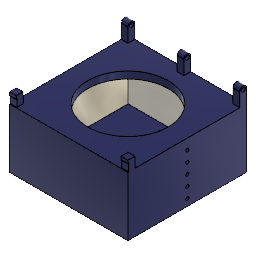
Final N95 UV Storage Container - Box v16 (Autodesk Fusion 360 design; units mm, degrees)
Autodesk Fusion 360 part; units mm, degrees
note: some values were not read from the file. Set by a fixed rule: which sketch regions a step uses.
sketch "Sketch1" plane through (0, 0, 0) normal (0, 0, 1) x (1, 0, 0)
  line L0 (0, 0) -> (170, 0)
  line L1 (170, 0) -> (170, 170)
  line L2 (170, 170) -> (0, 170)
  line L3 (0, 170) -> (0, 0)
  line L4 (0, 0) -> (85, 85)
  line L5 (87.25, 82.75) -> (82.75, 82.75)
  line L6 (82.75, 82.75) -> (82.75, 87.25)
  line L7 (82.75, 87.25) -> (87.25, 87.25)
  line L8 (87.25, 87.25) -> (87.25, 82.75)
  line L9 (87.25, 82.75) -> (82.75, 87.25) construction
  line L10 (82.75, 82.75) -> (87.25, 87.25) construction
  circle A0 centre (85, 85) radius 1.5
  point P0 (85, 85)
  dimension "d2" = 170
  dimension "d3" = 170
  dimension "d22" = 4.5
  dimension "d23" = 4.5
  dimension "d24" = 3
  dimension "d85" = 0
  dimension "d86" = 0
  dimension "d87" = 0
  dimension "d88" = 0
  dimension "d105" = 0
  dimension "d106" = 0
  dimension "d107" = 0
  dimension "d108" = 0
  dimension "d165" = 0
  dimension "d166" = 0
  dimension "d167" = 0
  dimension "d168" = 0
  dimension "d173" = 0
  dimension "d174" = 0
  dimension "d175" = 0
  dimension "d176" = 0
  dimension "d181" = 0
  dimension "d182" = 0
  dimension "d183" = 0
  constraint horizontal L0
  constraint vertical L1
  constraint horizontal L2
  constraint vertical L3
  constraint coincident L0.start L3.end
  constraint horizontal L5
  constraint perpendicular L5 L6
  constraint parallel L5 L7
  constraint parallel L6 L8
  constraint coincident L9 P0
  constraint coincident L10 P0
  constraint coincident P0 L4.end
  measures "d2" distance of L0.start L0.end
  measures "d3" distance of L0.start L2.end
  measures "d22" distance of L6.end L7.end
  measures "d23" distance of L5.end L6.end
  measures "d24" diameter of A0
extrude "Extrude1" add sketch "Sketch1" along normal blind 85 contours L0 L1 L2 L3 | L5 L6 L7 L8 | A0 makes body 1
shell "Shell1" thickness 10 removed faces 1 at (56.6667, 113.3333, 85) on bodies 1
extrude "Extrude3" cut sketch "Sketch1" along normal through all contours A0 bodies 1
extrude "Extrude4" cut sketch "Sketch1" along normal blind 10 and the other way blind -8 contours L5 L6 L7 L8 bodies 1
sketch "Sketch2" plane through (0, 0, 85) normal (0, 0, 1) x (-1, 0, 0)
  line L0 (-10, -160) -> (-160, -160)
  line L1 (-160, -160) -> (-160, -10)
  line L2 (-160, -10) -> (-10, -10)
  line L3 (-10, -10) -> (-10, -160)
  line L4 (0, -170) -> (0, 0)
  line L5 (0, 0) -> (-170, 0)
  line L6 (-170, 0) -> (-170, -170)
  line L7 (-170, -170) -> (0, -170)
  line L8 (0, -170) -> (-170, -170)
  line L9 (-170, -170) -> (-170, 0)
  line L10 (-170, 0) -> (0, 0)
  line L11 (0, 0) -> (0, -170)
  line L12 (0, 0) -> (-85, -85)
  circle A0 centre (-85, -85) radius 57.5
  dimension "d7" = 115
  constraint horizontal L8
  constraint vertical L9
  constraint horizontal L10
  constraint vertical L11
  constraint coincident L5.end L6.start
  constraint coincident L4.start L7.end
  constraint coincident L4.end L5.start
  constraint coincident L12.end A0.centre
  measures "d7" diameter of A0
extrude "Extrude2" add sketch "Sketch2" against normal blind 10 contours L0 L1 L2 L3 bodies 1
sketch "Sketch3" plane through (0, 0, 0) normal (-1, 0, 0) x (0, -1, 0)
  line L0 (-170, 0) -> (0, 0)
  line L1 (0, 0) -> (0, 85)
  line L2 (0, 85) -> (-170, 85)
  line L3 (-170, 85) -> (-170, 0)
  line L4 (-85, 85) -> (-85, 40)
  line L5 (-85, 85) -> (-85, 55)
  line L6 (-85, 85) -> (-85, 25)
  line L7 (-85, 85) -> (-85, 10)
  line L8 (-85, 85) -> (-85, 70)
  circle A0 centre (-85, 70) radius 2.25
  circle A1 centre (-85, 55) radius 2.25
  circle A2 centre (-85, 40) radius 2.25
  circle A3 centre (-85, 25) radius 2.25
  circle A4 centre (-85, 10) radius 2.25
  dimension "d10" = 45
  dimension "d69" = 30
  dimension "d70" = 60
  dimension "d71" = 75
  dimension "d72" = 15
  dimension "d73" = 4.5
  dimension "d74" = 4.5
  dimension "d75" = 4.5
  dimension "d76" = 4.5
  dimension "d77" = 4.5
  constraint midpoint L2 L4.start
  constraint perpendicular L0 L4
  constraint perpendicular L2 L5
  constraint perpendicular L2 L6
  constraint parallel L6 L7
  constraint parallel L6 L8
  constraint coincident L8.end A0.centre
  constraint coincident L5.end A1.centre
  constraint coincident L4.end A2.centre
  constraint coincident L6.end A3.centre
  constraint coincident L7.end A4.centre
  measures "d10" distance of L4.start L4.end
  measures "d69" distance of L4.start L5.end
  measures "d70" distance of L4.start L6.end
  measures "d71" distance of L4.start L7.end
  measures "d72" distance of L4.start L8.end
  measures "d73" diameter of A0
  measures "d74" diameter of A1
  measures "d75" diameter of A2
  measures "d76" diameter of A3
  measures "d77" diameter of A4
extrude "Extrude10" cut sketch "Sketch3" against normal blind 5 contours L4 L5 L6 L7 L8 A0 | L4 L5 L6 L7 L8 A0 | L4 L5 L6 L7 A1 | L4 L5 L6 L7 A1 | L4 L6 L7 A2 | L4 L6 L7 A2 | L6 L7 A3 | L6 L7 A3 | A4 bodies 1
ref_plane "WorkPlane1" through (85, 85, 42.5) normal (0, -1, 0) x (1, 0, 0)
sketch "Sketch4" plane through (85, 85, 55) normal (0, -1, 0) x (1, 0, 0)
  line L0 (-85, 10) -> (-94.9989, 10.1458)
  line L1 (-94.9989, 10.1458) -> (-95.1448, 0.1469)
  point P0 (-85, 10)
  dimension "d13" = 10
  dimension "d14" = 10
  constraint coincident P0 L0.start
  constraint perpendicular L0 L1
  measures "d13" distance of P0 L0.end
  measures "d14" distance of L0.end L1.end
pipe "Pipe1" [suppressed]
ref_plane "WorkPlane2" through (85, 85, 42.5) normal (-1, 0, 0) x (0, -1, 0)
mirror "Mirror2" about plane through (85, 85, 42.5) normal (-1, 0, 0) of "Extrude10"
mirror "Mirror1" [suppressed]
sketch "Sketch6" plane through (170, 0, 0) normal (1, 0, 0) x (0, 1, 0)
  line L0 (0, 0) -> (170, 0)
  line L1 (170, 0) -> (170, 85)
  line L2 (170, 85) -> (0, 85)
  line L3 (0, 85) -> (0, 0)
  line L4 (170, 85) -> (160, 85)
  line L5 (160, 85) -> (160, 105)
  line L6 (160, 105) -> (170, 105)
  line L7 (170, 105) -> (170, 85)
  circle A0 centre (165, 105) radius 5
  line L8 (0, 85) -> (10, 85)
  line L9 (10, 85) -> (10, 100)
  line L10 (10, 100) -> (0, 100)
  line L11 (0, 100) -> (0, 85)
  circle A1 centre (165, 105) radius 3
  line L12 (0, 100) -> (0, 95)
  line L13 (0, 95) -> (1.0607, 96.0607)
  line L14 (0, 95) -> (1.5, 95) construction
  line L15 (1.0607, 96.0607) -> (1.0607, 85)
  circle A2 centre (85, 40) radius 2.25
  circle A3 centre (85, 55) radius 2.25
  circle A4 centre (85, 25) radius 2.25
  circle A5 centre (85, 70) radius 2.25
  circle A6 centre (85, 10) radius 2.25
  dimension "d30" = 10
  dimension "d31" = 20
  dimension "d32" = 10
  dimension "d33" = 15
  dimension "d34" = 6
  dimension "d45" = 5
  dimension "d46" = 45
  dimension "d47" = 1.5
  constraint horizontal L4
  constraint vertical L5
  constraint horizontal L6
  constraint vertical L7
  constraint coincident L1.end L2.start
  constraint midpoint L6 A0.centre
  constraint coincident L5.end A0
  constraint horizontal L8
  constraint vertical L9
  constraint horizontal L10
  constraint vertical L11
  constraint coincident L2.end L3.start
  constraint concentric A0 A1
  constraint perpendicular L10 L12
  constraint horizontal L14
  constraint vertical L15
  constraint coincident L2 L15.end
  measures "d30" distance of L1.end L4.end
  measures "d31" distance of L1.end L6.end
  measures "d32" distance of L2.end L8.end
  measures "d33" distance of L2.end L10.end
  measures "d34" diameter of A1
  measures "d45" distance of L10.end L12.end
  measures "d46" angle of L13 L14
  measures "d47" distance of L12.end L13.end
extrude "Extrude5" add sketch "Sketch6" against normal blind 10 separate body contours L2 L4 L5 L7 A0 | L6 A0 A1 | L6 A0 A1 makes body 2
copy_body "CopyPasteBodies1" bodies 2 makes body 3
move_body "Move1" bodies 3 to x (1, 0, 0) y (0, 1, 0) z (0, 0, 1) at (-80, 0, 0)
copy_body "CopyPasteBodies2" bodies 2 makes body 4
move_body "Move2" bodies 4 to x (1, 0, 0) y (0, 1, 0) z (0, 0, 1) at (-160, 0, 0)
combine "Combine1" operation add target body 1 tool bodies 3 2 4
extrude "Extrude6" add sketch "Sketch6" against normal blind 10 separate body contours L2 L8 L9 L10 L11 L12 L13 L15 makes body 5
copy_body "CopyPasteBodies3" bodies 5 makes body 6
move_body "Move3" bodies 6 to x (1, 0, 0) y (0, 1, 0) z (0, 0, 1) at (-160, 0, 0)
sketch "Sketch9" plane through (0, 0, 8) normal (0, 0, 1) x (-1, 0, 0)
  circle A0 centre (-85, -85) radius 1.5
  line L0 (-87.25, -87.25) -> (-82.75, -87.25)
  line L1 (-82.75, -87.25) -> (-82.75, -82.75)
  line L2 (-82.75, -82.75) -> (-87.25, -82.75)
  line L3 (-87.25, -82.75) -> (-87.25, -87.25)
  line L4 (-82.75, -87.25) -> (-87.25, -87.25)
  line L5 (-87.25, -87.25) -> (-87.25, -82.75)
  line L6 (-87.25, -82.75) -> (-82.75, -82.75)
  line L7 (-82.75, -82.75) -> (-82.75, -87.25)
  line L8 (-86.725, -86.725) -> (-83.275, -86.725)
  line L9 (-83.275, -86.725) -> (-83.275, -83.275)
  line L10 (-83.275, -83.275) -> (-86.725, -83.275)
  line L11 (-86.725, -83.275) -> (-86.725, -86.725)
  line L12 (-86.725, -86.725) -> (-83.275, -83.275) construction
  line L13 (-83.275, -86.725) -> (-86.725, -83.275) construction
  circle A1 centre (-85, -85) radius 0.75
  point P0 (-85, -85)
  dimension "d48" = 3.45
  dimension "d49" = 3.45
  dimension "d50" = 1.5
  constraint horizontal L4
  constraint vertical L5
  constraint horizontal L6
  constraint vertical L7
  constraint coincident L2.end L3.start
  constraint coincident L0.end L1.start
  constraint horizontal L8
  constraint perpendicular L8 L9
  constraint parallel L8 L10
  constraint parallel L9 L11
  constraint coincident L12 P0
  constraint coincident L13 P0
  constraint coincident P0 A0.centre
  measures "d48" distance of L9.end L10.end
  measures "d49" distance of L8.end L9.end
  measures "d50" diameter of A1
extrude "Extrude8" add sketch "Sketch9" along normal blind 1 separate body contours A0 | L8 L9 L10 L11 | A1 makes body 7
ref_plane "WorkPlane3" through (85, 85, 8.5) normal (0, -1, 0) x (1, 0, 0)
sketch "Sketch10" plane through (85, 85, 8.5) normal (0, -1, 0) x (1, 0, 0)
  line L0 (0, 0.5) -> (-0.5, 0.5)
  line L1 (0, 0.5) -> (0.5, 0.5)
  line L2 (0, 0.5) -> (0, 1.5)
  line L3 (0, 0.5) -> (-1, 0.5)
  line L4 (0, 0.5) -> (1, 0.5)
  arc A0 (1, 0.5) -> (-1, 0.5) centre (0, 0.5) ccw
  line L5 (-1, 0.5) -> (1, 0.5)
  line L6 (1, 0.5) -> (1, 1.5)
  line L7 (1, 1.5) -> (-1, 1.5)
  line L8 (-1, 1.5) -> (-1, 0.5)
  dimension "d55" = 0.5
  dimension "d59" = 1
  dimension "d60" = 1
  dimension "d61" = 1
  dimension "d62" = 2
  dimension "d63" = 1
  constraint perpendicular L1 L2
  constraint perpendicular L2 L3
  constraint perpendicular L2 L4
  constraint coincident L2.end A0
  constraint horizontal L5
  constraint vertical L6
  constraint horizontal L7
  constraint vertical L8
  measures "d55" distance of L0.start L0.end
  measures "d59" distance of L0.start L2.end
  measures "d60" distance of L0.start L3.end
  measures "d61" distance of L0.start L4.end
  measures "d62" distance of L3.end L4.end
  measures "d63" distance of L3.end L7.end
revolve "Revolve1" [suppressed]
combine "Combine2" operation add target body 1 tool bodies 6 5
fillet "Fillet1" radius 0.2 2 edges at (165, 0, 95) (5, 0, 95) on bodies 1
extrude "Extrude9" add sketch "Sketch10" along normal blind 1 and the other way blind 1 bodies 7
fillet "Fillet2" radius 0.1 4 edges at (85, 86, 10) (86, 85, 10) (84, 85, 10) (85, 84, 10) on bodies 7
